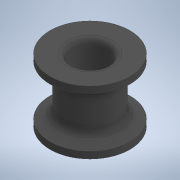
# Autodesk Inventor part: rolik
Saved by Autodesk Inventor 2020 (Build 240168000, 168)
## iProperties
Created: 2022-07-29
Part Number: rolik
Material: Типовые
Document SubType Name: Modeling
Designer: akapu
Density: 1 g/cm^3
Appearance: По умолчанию
Author: akapu
Autodesk Inventor part; units mm, degrees
ref_plane "YZ Plane" through (0, 0, 0) normal (1, 0, 0) x (0, 1, 0)
ref_plane "XZ Plane" through (0, 0, 0) normal (0, 1, 0) x (-1, 0, 0)
ref_plane "XY Plane" through (0, 0, 0) normal (0, 0, 1) x (1, 0, 0)
sketch "Эскиз1" plane through (0, 0, 0) normal (0, 1, 0) x (-1, 0, 0)
  circle A0 centre (0, 0) radius 2.7
  circle A1 centre (0, 0) radius 4
  dimension "d13" = 5.4
  dimension "d14" = 8
  constraints: 2 centre point, 1 coincident
  measures "d13" diameter of A0
  measures "d14" diameter of A1
extrude "Выдавливание1" add sketch "Эскиз1" along normal blind 9.5
sketch "Эскиз2" plane through (0, 9.5, 0) normal (0, 1, 0) x (1, 0, 0)
  circle A0 centre (0, 0) radius 1.6
  circle A1 centre (0, 0) radius 6
  circle A2 centre (0, 0) radius 2.7
  dimension "d15" = 12
  constraints: 3 centre point, 2 coincident
  measures "d15" diameter of A1
extrude "Выдавливание2" add sketch "Эскиз2" against normal blind 2 contours A1
sketch "Эскиз3" plane through (0, 0, 0) normal (0, -1, 0) x (1, 0, 0)
  circle A0 centre (0, 0) radius 2.7
  circle A1 centre (0, 0) radius 6
  constraints: 2 centre point, 2 coincident
extrude "Выдавливание3" add sketch "Эскиз3" against normal blind 2
sketch "Эскиз4" plane through (0, 0, 0) normal (0, 0, 1) x (1, 0, 0)
  line L0 (-2.7, 9.5) -> (2.7, 9.5) projected
  line L1 (0, 9.5) -> (0, 0)
  line L2 (6, 9.5) -> (6, 7.5) projected
  line L3 (-4, 7.5) -> (4, 7.5) projected
  line L4 (6, 8.5) -> (4, 7.5)
  line L5 (6, 8.5) -> (6, 7.5)
  line L6 (-6, 7.5) -> (6, 7.5) projected
  line L7 (4, 7.5) -> (6, 7.5)
  line L8 (6, 0) -> (6, 2) projected
  line L9 (6, 1) -> (4, 2)
  line L10 (4, 2) -> (6, 2)
  line L11 (6, 1) -> (6, 2)
  point P0 (5.5, 0)
  constraints: 14 end point, 3 midpoint, 2 collinear, 2 vertical, 1 horizontal
revolve "Вращение1" cut sketch "Эскиз4" angle 360 about axis through (0, 9.5, 0) along (0, -1, 0)
fillet "Сопряжение1" radius 1 4 edges at (0, 7.5, -4) (0, 7.5, 4) (0, 2, -4) (0, 2, 4)
fillet "Сопряжение2" radius 0.7 2 edges at (2.7, 0, 0) (2.7, 9.5, 0)
